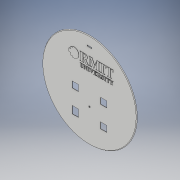
# Autodesk Inventor part: Cover
Saved by Autodesk Inventor 2018 (Build 220112000, 112)
## iProperties
Created: 2017-08-02
Part Number: Cover
Material: Generic
Document SubType Name: Modeling
Designer: Akram Al-Hourani
Density: 1 g/cm^3
Appearance: Default
Author: Akram Al-Hourani
Autodesk Inventor part; units mm, degrees
(part 1 of 2)
ref_plane "YZ Plane" through (0, 0, 0) normal (1, 0, 0) x (0, 1, 0)
ref_plane "XZ Plane" through (0, 0, 0) normal (0, 1, 0) x (-1, 0, 0)
ref_plane "XY Plane" through (0, 0, 0) normal (0, 0, 1) x (1, 0, 0)
sketch "Sketch1" plane through (0, 0, 0) normal (0, 0, 1) x (1, 0, 0)
  circle A0 centre (0, 0) radius 200
  circle A1 centre (0, 0) radius 194.25
  line L0 (-73, -28) -> (-47, -28)
  line L1 (-47, -28) -> (-47, -2)
  line L2 (-47, -2) -> (-73, -2)
  line L3 (-73, -2) -> (-73, -28)
  line L4 (-73, -28) -> (-47, -2) construction
  line L5 (-47, -28) -> (-73, -2) construction
  line L6 (47, -118) -> (73, -118)
  line L7 (73, -118) -> (73, -92)
  line L8 (73, -92) -> (47, -92)
  line L9 (47, -92) -> (47, -118)
  line L10 (47, -118) -> (73, -92) construction
  line L11 (73, -118) -> (47, -92) construction
  line L12 (47, -28) -> (73, -28)
  line L13 (73, -28) -> (73, -2)
  line L14 (73, -2) -> (47, -2)
  line L15 (47, -2) -> (47, -28)
  line L16 (47, -28) -> (73, -2) construction
  line L17 (73, -28) -> (47, -2) construction
  circle A2 centre (0, 0) radius 191.25
  line L18 (-103.842, 143.0933) -> (109.0153, 143.0933) construction
  line L19 (109.0153, 143.0933) -> (109.0153, 47.711) construction
  line L20 (109.0153, 47.711) -> (-103.842, 47.711) construction
  line L21 (-103.842, 47.711) -> (-103.842, 143.0933) construction
  line L22 (-70.0209, 127.2546) -> (-70.0209, 122.8615)
  line L23 (-70.0209, 122.8615) -> (-78.9535, 122.8615)
  line L24 (-78.9535, 122.8615) -> (-78.9535, 113.7335)
  line L25 (-78.9535, 113.7335) -> (-85.9337, 113.7335)
  line L26 (-85.9337, 113.7335) -> (-85.9337, 100.2125)
  line L27 (-85.9337, 100.2125) -> (-78.9535, 100.2125)
  line L28 (-78.9535, 100.2125) -> (-78.9535, 90.9382)
  line L29 (-78.9535, 90.9382) -> (-70.0209, 90.9382)
  line L30 (-70.0209, 90.9382) -> (-70.0209, 86.5939)
  line L31 (-70.0209, 86.5939) -> (-63.7485, 86.5939)
  line L32 (-70.0209, 127.2546) -> (-63.7485, 127.2546)
  arc A3 (-63.7485, 86.5939) -> (-63.7485, 127.2546) centre (-64.7193, 106.9242) ccw
  line L33 (-41.3776, 125.1847) -> (92.2863, 125.1847) construction
  line L34 (92.2863, 125.1847) -> (92.2863, 80.3812) construction
  line L35 (92.2863, 80.3812) -> (-41.3776, 80.3812) construction
  line L36 (-41.3776, 80.3812) -> (-41.3776, 125.1847) construction
  line L37 (-40.2575, 83.3681) -> (113.1946, 83.3681) construction
  line L38 (113.1946, 83.3681) -> (113.1946, 53.1257) construction
  line L39 (113.1946, 53.1257) -> (-40.2575, 53.1257) construction
  line L40 (-40.2575, 53.1257) -> (-40.2575, 83.3681) construction
  line L41 (-10, 156.8645) -> (10, 156.8645)
  line L42 (10, 156.8645) -> (10, 161.8645)
  line L43 (10, 161.8645) -> (-10, 161.8645)
  line L44 (-10, 161.8645) -> (-10, 156.8645)
  line L45 (-10, 156.8645) -> (10, 161.8645) construction
  line L46 (10, 156.8645) -> (-10, 161.8645) construction
  line L47 (-60, -15) -> (60, -105) construction
  line L48 (-60, -15) -> (60, -15) construction
  line L49 (60, -15) -> (60, -105) construction
  line L50 (60, -105) -> (-60, -105) construction
  line L51 (-60, -105) -> (-60, -15) construction
  line L52 (-73, -118) -> (-47, -118)
  line L53 (-47, -118) -> (-47, -92)
  line L54 (-47, -92) -> (-73, -92)
  line L55 (-73, -92) -> (-73, -118)
  line L56 (-73, -118) -> (-47, -92) construction
  line L57 (-47, -118) -> (-73, -92) construction
  line L58 (60, -15) -> (-60, -105) construction
  line L59 (-73, -118) -> (-47, -118)
  line L60 (-47, -118) -> (-47, -123)
  line L61 (-47, -123) -> (-73, -123)
  line L62 (-73, -123) -> (-73, -118)
  circle A4 centre (0, -60) radius 1
  circle A5 centre (0, -60) radius 3
  line L63 (-27.3375, 106.1406) -> (-27.3375, 96.3326)
  spline S0 degree 2 poles (-27.3375, 96.3326) (-27.3375, 93.4731) (-26.6513, 92.0148) (-24.8784, 91.1283) (-22.4764, 91.1283) knots 0 0 0 1 2 3 3 3
  line L64 (-22.4764, 91.1283) -> (-22.4764, 90.1847)
  line L65 (-22.4764, 90.1847) -> (-40.4053, 90.1847)
  line L66 (-40.4053, 90.1847) -> (-40.4053, 91.1283)
  spline S1 degree 2 poles (-40.4053, 91.1283) (-37.9748, 91.1283) (-36.2305, 92.0434) (-35.5442, 93.4731) (-35.5442, 96.3326) knots 0 0 0 1 2 3 3 3
  line L67 (-35.5442, 96.3326) -> (-35.5442, 119.0368)
  spline S2 degree 2 poles (-35.5442, 119.0368) (-35.5442, 121.8963) (-36.2305, 123.3546) (-38.0034, 124.2411) (-40.4053, 124.2411) knots 0 0 0 1 2 3 3 3
  line L68 (-40.4053, 124.2411) -> (-40.4053, 125.1847)
  line L69 (-40.4053, 125.1847) -> (-24.1349, 125.1847)
  spline S3 degree 2 poles (-24.1349, 125.1847) (-17.7869, 125.1847) (-11.8964, 123.4404) (-8.179, 118.7223) (-8.179, 115.5483) knots 0 0 0 1 2 3 3 3
  spline S4 degree 2 poles (-8.179, 115.5483) (-8.179, 111.6594) (-10.9813, 109.143) knots 0 0 0 1 1 1
  spline S5 degree 2 poles (-10.9813, 109.143) (-12.7542, 107.5417) (-15.9568, 106.7411) knots 0 0 0 1 1 1
  line L70 (-15.9568, 106.7411) -> (-7.55, 94.8743)
  spline S6 degree 2 poles (-7.55, 94.8743) (-5.8915, 92.5581) (-5.1766, 92.0148) knots 0 0 0 1 1 1
  spline S7 degree 2 poles (-5.1766, 92.0148) (-4.1186, 91.2141) (-2.7174, 91.1283) knots 0 0 0 1 1 1
  line L71 (-2.7174, 91.1283) -> (-2.7174, 90.1847)
  line L72 (-2.7174, 90.1847) -> (-13.755, 90.1847)
  line L73 (-13.755, 90.1847) -> (-25.05, 106.1406)
  line L74 (-25.05, 106.1406) -> (-27.3375, 106.1406)
  line L75 (-27.3375, 123.2975) -> (-27.3375, 107.9707)
  line L76 (-27.3375, 107.9707) -> (-25.8792, 107.9707)
  spline S8 degree 2 poles (-25.8792, 107.9707) (-22.2763, 107.9707) (-18.7019, 109.286) (-16.6717, 112.7174) (-16.6717, 115.4911) knots 0 0 0 1 2 3 3 3
  spline S9 degree 2 poles (-16.6717, 115.4911) (-16.6717, 119.4658) (-20.4176, 123.2975) (-24.5638, 123.2975) knots 0 0 0 1 2 2 2
  line L77 (-24.5638, 123.2975) -> (-27.3375, 123.2975)
  line L78 (22.017, 102.1659) -> (31.5105, 125.1847)
  line L79 (31.5105, 125.1847) -> (45.7221, 125.1847)
  line L80 (45.7221, 125.1847) -> (45.7221, 124.2411)
  line L81 (45.7221, 124.2411) -> (44.5783, 124.2411)
  spline S10 degree 2 poles (44.5783, 124.2411) (43.0342, 124.2411) (42.1192, 123.6978) knots 0 0 0 1 1 1
  spline S11 degree 2 poles (42.1192, 123.6978) (41.4615, 123.3261) (41.0897, 122.4682) knots 0 0 0 1 1 1
  spline S12 degree 2 poles (41.0897, 122.4682) (40.8038, 121.8677) (40.8038, 119.237) knots 0 0 0 1 1 1
  line L82 (40.8038, 119.237) -> (40.8038, 96.161)
  spline S13 degree 2 poles (40.8038, 96.161) (40.8038, 93.4731) (41.3757, 92.1292) (43.12, 91.1283) (44.5783, 91.1283) knots 0 0 0 1 2 3 3 3
  line L83 (44.5783, 91.1283) -> (45.7221, 91.1283)
  line L84 (45.7221, 91.1283) -> (45.7221, 90.1847)
  line L85 (45.7221, 90.1847) -> (27.4786, 90.1847)
  line L86 (27.4786, 90.1847) -> (27.4786, 91.1283)
  line L87 (27.4786, 91.1283) -> (28.6224, 91.1283)
  spline S14 degree 2 poles (28.6224, 91.1283) (30.1665, 91.1283) (31.0816, 91.6716) knots 0 0 0 1 1 1
  spline S15 degree 2 poles (31.0816, 91.6716) (31.7393, 92.0434) (32.111, 92.9012) knots 0 0 0 1 1 1
  spline S16 degree 2 poles (32.111, 92.9012) (32.3969, 93.5303) (32.3969, 96.161) knots 0 0 0 1 1 1
  line L88 (32.3969, 96.161) -> (32.3969, 122.0965)
  line L89 (32.3969, 122.0965) -> (18.986, 90.1847)
  line L90 (18.986, 90.1847) -> (18.3569, 90.1847)
  line L91 (18.3569, 90.1847) -> (4.7172, 121.8677)
  line L92 (4.7172, 121.8677) -> (4.7172, 97.219)
  spline S17 degree 2 poles (4.7172, 97.219) (4.7172, 94.6455) (4.8602, 94.045) knots 0 0 0 1 1 1
  spline S18 degree 2 poles (4.8602, 94.045) (5.1747, 92.7582) (7.4337, 91.1283) (9.8357, 91.1283) knots 0 0 0 1 2 2 2
  line L93 (9.8357, 91.1283) -> (9.8357, 90.1847)
  line L94 (9.8357, 90.1847) -> (-2.1741, 90.1847)
  line L95 (-2.1741, 90.1847) -> (-2.1741, 91.1283)
  line L96 (-2.1741, 91.1283) -> (-1.8024, 91.1283)
  spline S19 degree 2 poles (-1.8024, 91.1283) (-0.63, 91.0997) (1.3716, 91.9004) (2.401, 93.2729) (2.687, 94.4739) knots 0 0 0 1 2 3 3 3
  spline S20 degree 2 poles (2.687, 94.4739) (2.7442, 94.7599) (2.7442, 97.1332) knots 0 0 0 1 1 1
  line L97 (2.7442, 97.1332) -> (2.7442, 119.237)
  spline S21 degree 2 poles (2.7442, 119.237) (2.7442, 121.8963) (2.1723, 123.2403) (0.428, 124.2411) (-1.0589, 124.2411) knots 0 0 0 1 2 3 3 3
  line L98 (-1.0589, 124.2411) -> (-2.1741, 124.2411)
  line L99 (-2.1741, 124.2411) -> (-2.1741, 125.1847)
  line L100 (-2.1741, 125.1847) -> (12.1804, 125.1847)
  line L101 (12.1804, 125.1847) -> (22.017, 102.1659)
  line L102 (65.9958, 91.1283) -> (65.9958, 90.1847)
  line L103 (65.9958, 90.1847) -> (47.7523, 90.1847)
  line L104 (47.7523, 90.1847) -> (47.7523, 91.1283)
  line L105 (47.7523, 91.1283) -> (48.9247, 91.1283)
  spline S22 degree 2 poles (48.9247, 91.1283) (50.4402, 91.1283) (51.3553, 91.6716) knots 0 0 0 1 1 1
  spline S23 degree 2 poles (51.3553, 91.6716) (52.013, 92.0434) (52.3847, 92.9012) knots 0 0 0 1 1 1
  spline S24 degree 2 poles (52.3847, 92.9012) (52.6706, 93.5303) (52.6706, 96.161) knots 0 0 0 1 1 1
  line L106 (52.6706, 96.161) -> (52.6706, 119.2084)
  spline S25 degree 2 poles (52.6706, 119.2084) (52.6706, 121.8963) (52.0987, 123.2403) (50.383, 124.2411) (48.9247, 124.2411) knots 0 0 0 1 2 3 3 3
  line L107 (48.9247, 124.2411) -> (47.7523, 124.2411)
  line L108 (47.7523, 124.2411) -> (47.7523, 125.1847)
  line L109 (47.7523, 125.1847) -> (65.9958, 125.1847)
  line L110 (65.9958, 125.1847) -> (65.9958, 124.2411)
  line L111 (65.9958, 124.2411) -> (64.852, 124.2411)
  spline S26 degree 2 poles (64.852, 124.2411) (63.3365, 124.2411) (62.4214, 123.6978) knots 0 0 0 1 1 1
  spline S27 degree 2 poles (62.4214, 123.6978) (61.7352, 123.3261) (61.3634, 122.4682) knots 0 0 0 1 1 1
  spline S28 degree 2 poles (61.3634, 122.4682) (61.0775, 121.8391) (61.0775, 119.2084) knots 0 0 0 1 1 1
  line L112 (61.0775, 119.2084) -> (61.0775, 96.161)
  spline S29 degree 2 poles (61.0775, 96.161) (61.0775, 93.4731) (61.678, 92.1292) (63.3937, 91.1283) (64.852, 91.1283) knots 0 0 0 1 2 3 3 3
  line L113 (64.852, 91.1283) -> (65.9958, 91.1283)
  line L114 (100.6527, 125.1847) -> (100.6527, 115.7198)
  line L115 (100.6527, 115.7198) -> (99.709, 115.7198)
  spline S30 degree 2 poles (99.709, 115.7198) (98.8798, 119.0082) (96.8781, 121.8677) (95.1339, 122.7256) knots 0 0 0 1 2 2 2
  spline S31 degree 2 poles (95.1339, 122.7256) (94.1616, 123.1831) (91.7025, 123.1831) knots 0 0 0 1 1 1
  line L116 (91.7025, 123.1831) -> (89.1004, 123.1831)
  line L117 (89.1004, 123.1831) -> (89.1004, 96.161)
  spline S32 degree 2 poles (89.1004, 96.161) (89.1004, 93.4731) (89.7009, 92.1292) (91.4165, 91.1283) (92.9035, 91.1283) knots 0 0 0 1 2 3 3 3
  line L118 (92.9035, 91.1283) -> (94.0759, 91.1283)
  line L119 (94.0759, 91.1283) -> (94.0759, 90.1847)
  line L120 (94.0759, 90.1847) -> (75.7752, 90.1847)
  line L121 (75.7752, 90.1847) -> (75.7752, 91.1283)
  line L122 (75.7752, 91.1283) -> (76.919, 91.1283)
  spline S33 degree 2 poles (76.919, 91.1283) (78.4345, 91.1283) (79.3496, 91.6716) knots 0 0 0 1 1 1
  spline S34 degree 2 poles (79.3496, 91.6716) (80.0358, 92.0434) (80.4076, 92.9012) knots 0 0 0 1 1 1
  spline S35 degree 2 poles (80.4076, 92.9012) (80.6935, 93.5303) (80.6935, 96.161) knots 0 0 0 1 1 1
  line L123 (80.6935, 96.161) -> (80.6935, 123.1831)
  line L124 (80.6935, 123.1831) -> (78.1486, 123.1831)
  spline S36 degree 2 poles (78.1486, 123.1831) (74.6028, 123.1831) (73.0015, 121.6962) knots 0 0 0 1 1 1
  spline S37 degree 2 poles (73.0015, 121.6962) (70.7425, 119.5801) (70.142, 115.7198) knots 0 0 0 1 1 1
  line L125 (70.142, 115.7198) -> (69.1984, 115.7198)
  line L126 (69.1984, 115.7198) -> (69.1984, 125.1847)
  line L127 (69.1984, 125.1847) -> (100.6527, 125.1847)
  line L128 (-39.7305, 83.0249) -> (-31.9854, 83.0249)
  line L129 (-31.9854, 83.0249) -> (-31.9854, 82.6205)
  line L130 (-31.9854, 82.6205) -> (-32.3776, 82.6205)
  spline S38 degree 2 poles (-32.3776, 82.6205) (-33.2477, 82.6205) (-33.8972, 82.2529) (-34.1791, 81.6156) (-34.1791, 80.3289) knots 0 0 0 1 2 3 3 3
  line L131 (-34.1791, 80.3289) -> (-34.1791, 72.9882)
  spline S39 degree 2 poles (-34.1791, 72.9882) (-34.1791, 70.9784) (-33.5663, 69.6671) (-32.1815, 68.8093) (-31.1153, 68.8093) knots 0 0 0 1 2 3 3 3
  spline S40 degree 2 poles (-31.1153, 68.8093) (-29.9021, 68.8093) (-28.1864, 69.8999) (-27.3286, 71.824) (-27.3286, 74.2137) knots 0 0 0 1 2 3 3 3
  line L132 (-27.3286, 74.2137) -> (-27.3286, 80.3289)
  spline S41 degree 2 poles (-27.3286, 80.3289) (-27.3286, 81.3338) (-27.7452, 82.2039) (-28.0639, 82.3632) knots 0 0 0 1 2 2 2
  spline S42 degree 2 poles (-28.0639, 82.3632) (-28.5663, 82.6205) (-29.4732, 82.6205) knots 0 0 0 1 1 1
  line L133 (-29.4732, 82.6205) -> (-29.4732, 83.0249)
  line L134 (-29.4732, 83.0249) -> (-24.2893, 83.0249)
  line L135 (-24.2893, 83.0249) -> (-24.2893, 82.6205)
  line L136 (-24.2893, 82.6205) -> (-24.5957, 82.6205)
  spline S43 degree 2 poles (-24.5957, 82.6205) (-25.233, 82.6205) (-26.0663, 82.1058) (-26.2501, 81.6034) knots 0 0 0 1 2 2 2
  spline S44 degree 2 poles (-26.2501, 81.6034) (-26.3972, 81.248) (-26.3972, 80.3289) knots 0 0 0 1 1 1
  line L137 (-26.3972, 80.3289) -> (-26.3972, 74.6303)
  spline S45 degree 2 poles (-26.3972, 74.6303) (-26.3972, 71.9955) (-27.0957, 69.6549) (-29.7918, 67.6818) (-32.1325, 67.6818) knots 0 0 0 1 2 3 3 3
  spline S46 degree 2 poles (-32.1325, 67.6818) (-34.081, 67.6818) (-35.1349, 68.1965) knots 0 0 0 1 1 1
  spline S47 degree 2 poles (-35.1349, 68.1965) (-36.581, 68.9073) (-37.782, 71.1254) (-37.782, 72.9882) knots 0 0 0 1 2 2 2
  line L138 (-37.782, 72.9882) -> (-37.782, 80.3289)
  spline S48 degree 2 poles (-37.782, 80.3289) (-37.782, 81.6279) (-38.0639, 82.2529) (-38.7746, 82.6328) (-39.7305, 82.6205) knots 0 0 0 1 2 3 3 3
  line L139 (-39.7305, 82.6205) -> (-39.7305, 83.0249)
  line L140 (-18.2599, 83.0249) -> (-10.858, 73.7235)
  line L141 (-10.858, 73.7235) -> (-10.858, 80.1696)
  spline S49 degree 2 poles (-10.858, 80.1696) (-10.858, 81.5176) (-11.2501, 81.9955) knots 0 0 0 1 1 1
  spline S50 degree 2 poles (-11.2501, 81.9955) (-11.7771, 82.645) (-13.0271, 82.6205) knots 0 0 0 1 1 1
  line L142 (-13.0271, 82.6205) -> (-13.0271, 83.0249)
  line L143 (-13.0271, 83.0249) -> (-8.0639, 83.0249)
  line L144 (-8.0639, 83.0249) -> (-8.0639, 82.6205)
  spline S51 degree 2 poles (-8.0639, 82.6205) (-9.0197, 82.498) (-9.6692, 82.1058) (-10.0369, 81.2357) (-10.0369, 80.1696) knots 0 0 0 1 2 3 3 3
  line L145 (-10.0369, 80.1696) -> (-10.0369, 67.6818)
  line L146 (-10.0369, 67.6818) -> (-10.4168, 67.6818)
  line L147 (-10.4168, 67.6818) -> (-20.5639, 80.1818)
  line L148 (-20.5639, 80.1818) -> (-20.5639, 70.6352)
  spline S52 degree 2 poles (-20.5639, 70.6352) (-20.5639, 69.3362) (-19.3751, 68.4294) (-18.6153, 68.4294) knots 0 0 0 1 2 2 2
  line L149 (-18.6153, 68.4294) -> (-18.2599, 68.4294)
  line L150 (-18.2599, 68.4294) -> (-18.2599, 68.0249)
  line L151 (-18.2599, 68.0249) -> (-23.5908, 68.0249)
  line L152 (-23.5908, 68.0249) -> (-23.5908, 68.4294)
  spline S53 degree 2 poles (-23.5908, 68.4294) (-22.3531, 68.4416) (-21.3727, 69.4343) (-21.3727, 70.6352) knots 0 0 0 1 2 2 2
  line L153 (-21.3727, 70.6352) -> (-21.3727, 81.2235)
  line L154 (-21.3727, 81.2235) -> (-21.6913, 81.6156)
  spline S54 degree 2 poles (-21.6913, 81.6156) (-22.1692, 82.2161) (-22.8923, 82.596) (-23.5786, 82.6205) knots 0 0 0 1 2 2 2
  line L155 (-23.5786, 82.6205) -> (-23.5786, 83.0249)
  line L156 (-23.5786, 83.0249) -> (-18.2599, 83.0249)
  line L157 (0.7352, 68.4294) -> (0.7352, 68.0249)
  line L158 (0.7352, 68.0249) -> (-7.0835, 68.0249)
  line L159 (-7.0835, 68.0249) -> (-7.0835, 68.4294)
  line L160 (-7.0835, 68.4294) -> (-6.581, 68.4294)
  spline S55 degree 2 poles (-6.581, 68.4294) (-5.9315, 68.4294) (-5.5393, 68.6622) knots 0 0 0 1 1 1
  spline S56 degree 2 poles (-5.5393, 68.6622) (-5.2575, 68.8215) (-5.0982, 69.1892) knots 0 0 0 1 1 1
  spline S57 degree 2 poles (-5.0982, 69.1892) (-4.9756, 69.4588) (-4.9756, 70.5862) knots 0 0 0 1 1 1
  line L161 (-4.9756, 70.5862) -> (-4.9756, 80.4637)
  spline S58 degree 2 poles (-4.9756, 80.4637) (-4.9756, 81.6156) (-5.2207, 82.1916) (-5.956, 82.6205) (-6.581, 82.6205) knots 0 0 0 1 2 3 3 3
  line L162 (-6.581, 82.6205) -> (-7.0835, 82.6205)
  line L163 (-7.0835, 82.6205) -> (-7.0835, 83.0249)
  line L164 (-7.0835, 83.0249) -> (0.7352, 83.0249)
  line L165 (0.7352, 83.0249) -> (0.7352, 82.6205)
  line L166 (0.7352, 82.6205) -> (0.245, 82.6205)
  spline S59 degree 2 poles (0.245, 82.6205) (-0.4045, 82.6205) (-0.7967, 82.3877) knots 0 0 0 1 1 1
  spline S60 degree 2 poles (-0.7967, 82.3877) (-1.0908, 82.2284) (-1.2501, 81.8607) knots 0 0 0 1 1 1
  spline S61 degree 2 poles (-1.2501, 81.8607) (-1.3727, 81.5911) (-1.3727, 80.4637) knots 0 0 0 1 1 1
  line L167 (-1.3727, 80.4637) -> (-1.3727, 70.5862)
  spline S62 degree 2 poles (-1.3727, 70.5862) (-1.3727, 69.4343) (-1.1153, 68.8583) (-0.38, 68.4294) (0.245, 68.4294) knots 0 0 0 1 2 3 3 3
  line L168 (0.245, 68.4294) -> (0.7352, 68.4294)
  line L169 (17.4141, 83.0249) -> (17.4141, 82.6205)
  spline S63 degree 2 poles (17.4141, 82.6205) (16.593, 82.4857) (15.9558, 81.7504) knots 0 0 0 1 1 1
  spline S64 degree 2 poles (15.9558, 81.7504) (15.4901, 81.1867) (14.5709, 79.1401) knots 0 0 0 1 1 1
  line L170 (14.5709, 79.1401) -> (9.3994, 67.6818)
  line L171 (9.3994, 67.6818) -> (9.0317, 67.6818)
  line L172 (9.0317, 67.6818) -> (3.9092, 79.6181)
  spline S65 degree 2 poles (3.9092, 79.6181) (2.9778, 81.7749) (2.3528, 82.5225) (1.4827, 82.6205) knots 0 0 0 1 2 2 2
  line L173 (1.4827, 82.6205) -> (1.4827, 83.0249)
  line L174 (1.4827, 83.0249) -> (8.6518, 83.0249)
  line L175 (8.6518, 83.0249) -> (8.6518, 82.6205)
  line L176 (8.6518, 82.6205) -> (8.4067, 82.6205)
  spline S66 degree 2 poles (8.4067, 82.6205) (7.4386, 82.6205) (7.0832, 82.3754) knots 0 0 0 1 1 1
  spline S67 degree 2 poles (7.0832, 82.3754) (6.8259, 82.2039) (6.8259, 81.8852) knots 0 0 0 1 1 1
  spline S68 degree 2 poles (6.8259, 81.8852) (6.8259, 81.6892) (6.9974, 81.1499) (7.5121, 79.9612) knots 0 0 0 1 2 2 2
  line L177 (7.5121, 79.9612) -> (10.7107, 72.498)
  line L178 (10.7107, 72.498) -> (13.6763, 79.1524)
  spline S69 degree 2 poles (13.6763, 79.1524) (14.2033, 80.3534) (14.4484, 81.1622) (14.4484, 81.4563) knots 0 0 0 1 2 2 2
  spline S70 degree 2 poles (14.4484, 81.4563) (14.4484, 81.7872) (14.093, 82.3019) (13.7499, 82.4367) knots 0 0 0 1 2 2 2
  spline S71 degree 2 poles (13.7499, 82.4367) (13.2719, 82.6205) (12.4876, 82.6205) knots 0 0 0 1 1 1
  line L179 (12.4876, 82.6205) -> (12.4876, 83.0249)
  line L180 (12.4876, 83.0249) -> (17.4141, 83.0249)
  line L181 (23.8111, 82.1671) -> (23.8111, 76.0642)
  line L182 (23.8111, 76.0642) -> (24.1175, 76.0642)
  spline S72 degree 2 poles (24.1175, 76.0642) (25.5513, 76.0642) (26.8381, 77.8534) (27.0219, 79.6058) knots 0 0 0 1 2 2 2
  line L183 (27.0219, 79.6058) -> (27.4263, 79.6058)
  line L184 (27.4263, 79.6058) -> (27.4263, 71.7504)
  line L185 (27.4263, 71.7504) -> (27.0219, 71.7504)
  spline S73 degree 2 poles (27.0219, 71.7504) (26.8871, 73.0372) (26.0293, 74.6671) (24.8896, 75.2308) (23.8111, 75.2308) knots 0 0 0 1 2 3 3 3
  line L186 (23.8111, 75.2308) -> (23.8111, 71.0029)
  spline S74 degree 2 poles (23.8111, 71.0029) (23.8111, 69.7651) (24.0195, 69.2137) (24.5955, 68.8583) (25.245, 68.8583) knots 0 0 0 1 2 3 3 3
  line L187 (25.245, 68.8583) -> (26.1396, 68.8583)
  spline S75 degree 2 poles (26.1396, 68.8583) (28.2474, 68.8583) (30.7842, 70.8068) (31.3357, 72.7921) knots 0 0 0 1 2 2 2
  line L188 (31.3357, 72.7921) -> (31.7401, 72.7921)
  line L189 (31.7401, 72.7921) -> (31.066, 68.0249)
  line L190 (31.066, 68.0249) -> (18.1004, 68.0249)
  line L191 (18.1004, 68.0249) -> (18.1004, 68.4294)
  line L192 (18.1004, 68.4294) -> (18.6028, 68.4294)
  spline S76 degree 2 poles (18.6028, 68.4294) (19.2523, 68.4294) (19.6445, 68.6622) knots 0 0 0 1 1 1
  spline S77 degree 2 poles (19.6445, 68.6622) (19.9263, 68.8215) (20.0857, 69.1892) knots 0 0 0 1 1 1
  spline S78 degree 2 poles (20.0857, 69.1892) (20.2082, 69.4588) (20.2082, 70.5862) knots 0 0 0 1 1 1
  line L193 (20.2082, 70.5862) -> (20.2082, 80.4637)
  spline S79 degree 2 poles (20.2082, 80.4637) (20.2082, 81.4808) (20.1592, 81.7137) knots 0 0 0 1 1 1
  spline S80 degree 2 poles (20.1592, 81.7137) (20.0366, 82.1058) (19.7425, 82.3142) knots 0 0 0 1 1 1
  spline S81 degree 2 poles (19.7425, 82.3142) (19.3259, 82.6205) (18.6028, 82.6205) knots 0 0 0 1 1 1
  line L194 (18.6028, 82.6205) -> (18.1004, 82.6205)
  line L195 (18.1004, 82.6205) -> (18.1004, 83.0249)
  line L196 (18.1004, 83.0249) -> (30.6616, 83.0249)
  line L197 (30.6616, 83.0249) -> (30.6616, 78.5887)
  line L198 (30.6616, 78.5887) -> (30.2572, 78.5887)
  spline S82 degree 2 poles (30.2572, 78.5887) (29.9386, 80.2186) (28.7621, 81.6401) (27.6959, 81.971) knots 0 0 0 1 2 2 2
  spline S83 degree 2 poles (27.6959, 81.971) (27.0832, 82.1671) (25.3675, 82.1671) knots 0 0 0 1 1 1
  line L199 (25.3675, 82.1671) -> (23.8111, 82.1671)
  line L200 (38.7744, 74.8632) -> (38.7744, 70.6598)
  spline S84 degree 2 poles (38.7744, 70.6598) (38.7744, 69.4343) (39.0685, 68.8093) (39.8283, 68.4294) (40.8577, 68.4294) knots 0 0 0 1 2 3 3 3
  line L201 (40.8577, 68.4294) -> (40.8577, 68.0249)
  line L202 (40.8577, 68.0249) -> (33.1739, 68.0249)
  line L203 (33.1739, 68.0249) -> (33.1739, 68.4294)
  spline S85 degree 2 poles (33.1739, 68.4294) (34.2156, 68.4294) (34.9631, 68.8215) (35.2572, 69.4343) (35.2572, 70.6598) knots 0 0 0 1 2 3 3 3
  line L204 (35.2572, 70.6598) -> (35.2572, 80.3901)
  spline S86 degree 2 poles (35.2572, 80.3901) (35.2572, 81.6156) (34.9631, 82.2406) (34.2033, 82.6205) (33.1739, 82.6205) knots 0 0 0 1 2 3 3 3
  line L205 (33.1739, 82.6205) -> (33.1739, 83.0249)
  line L206 (33.1739, 83.0249) -> (40.1469, 83.0249)
  spline S87 degree 2 poles (40.1469, 83.0249) (42.8675, 83.0249) (45.392, 82.2774) (46.9852, 80.2553) (46.9852, 78.895) knots 0 0 0 1 2 3 3 3
  spline S88 degree 2 poles (46.9852, 78.895) (46.9852, 77.2284) (45.7842, 76.1499) knots 0 0 0 1 1 1
  spline S89 degree 2 poles (45.7842, 76.1499) (45.0244, 75.4637) (43.6518, 75.1205) knots 0 0 0 1 1 1
  line L207 (43.6518, 75.1205) -> (47.2548, 70.0348)
  spline S90 degree 2 poles (47.2548, 70.0348) (47.9656, 69.0421) (48.2719, 68.8093) knots 0 0 0 1 1 1
  spline S91 degree 2 poles (48.2719, 68.8093) (48.7254, 68.4661) (49.3259, 68.4294) knots 0 0 0 1 1 1
  line L208 (49.3259, 68.4294) -> (49.3259, 68.0249)
  line L209 (49.3259, 68.0249) -> (44.5955, 68.0249)
  line L210 (44.5955, 68.0249) -> (39.7548, 74.8632)
  line L211 (39.7548, 74.8632) -> (38.7744, 74.8632)
  line L212 (38.7744, 82.2161) -> (38.7744, 75.6475)
  line L213 (38.7744, 75.6475) -> (39.3994, 75.6475)
  spline S92 degree 2 poles (39.3994, 75.6475) (40.9435, 75.6475) (42.4754, 76.2112) (43.3455, 77.6818) (43.3455, 78.8705) knots 0 0 0 1 2 3 3 3
  spline S93 degree 2 poles (43.3455, 78.8705) (43.3455, 80.574) (41.7401, 82.2161) (39.9631, 82.2161) knots 0 0 0 1 2 2 2
  line L214 (39.9631, 82.2161) -> (38.7744, 82.2161)
  line L215 (59.7548, 83.3681) -> (59.8773, 78.3681)
  line L216 (59.8773, 78.3681) -> (59.4239, 78.3681)
  spline S94 degree 2 poles (59.4239, 78.3681) (59.1053, 80.2431) (56.5808, 82.5348) (55.1224, 82.5348) knots 0 0 0 1 2 2 2
  spline S95 degree 2 poles (55.1224, 82.5348) (53.995, 82.5348) (52.6714, 81.3338) (52.6714, 80.5495) knots 0 0 0 1 2 2 2
  spline S96 degree 2 poles (52.6714, 80.5495) (52.6714, 80.047) (52.9043, 79.6671) knots 0 0 0 1 1 1
  spline S97 degree 2 poles (52.9043, 79.6671) (53.2229, 79.1401) (53.9337, 78.6377) knots 0 0 0 1 1 1
  spline S98 degree 2 poles (53.9337, 78.6377) (54.4607, 78.27) (56.3479, 77.3387) knots 0 0 0 1 1 1
  spline S99 degree 2 poles (56.3479, 77.3387) (58.9827, 76.0519) (59.9018, 74.8999) knots 0 0 0 1 1 1
  spline S100 degree 2 poles (59.9018, 74.8999) (60.8087, 73.748) (60.8087, 72.2651) knots 0 0 0 1 1 1
  spline S101 degree 2 poles (60.8087, 72.2651) (60.8087, 70.3901) (57.8798, 67.6818) (55.6126, 67.6818) knots 0 0 0 1 2 2 2
  spline S102 degree 2 poles (55.6126, 67.6818) (54.9018, 67.6818) (53.6396, 67.9637) (52.6959, 68.3681) knots 0 0 0 1 2 2 2
  spline S103 degree 2 poles (52.6959, 68.3681) (52.1567, 68.5887) (51.8136, 68.5887) knots 0 0 0 1 1 1
  spline S104 degree 2 poles (51.8136, 68.5887) (51.5317, 68.5887) (50.8822, 68.1352) (50.6861, 67.6818) knots 0 0 0 1 2 2 2
  line L217 (50.6861, 67.6818) -> (50.2817, 67.6818)
  line L218 (50.2817, 67.6818) -> (50.2817, 73.3436)
  line L219 (50.2817, 73.3436) -> (50.6861, 73.3436)
  spline S105 degree 2 poles (50.6861, 73.3436) (51.1763, 70.9539) (53.9582, 68.4539) (55.5636, 68.4539) knots 0 0 0 1 2 2 2
  spline S106 degree 2 poles (55.5636, 68.4539) (56.8013, 68.4539) (58.2719, 69.8019) (58.2719, 70.6965) knots 0 0 0 1 2 2 2
  spline S107 degree 2 poles (58.2719, 70.6965) (58.2719, 71.2235) (57.7082, 72.2284) (56.5562, 73.123) (55.0857, 73.8338) knots 0 0 0 1 2 3 3 3
  spline S108 degree 2 poles (55.0857, 73.8338) (53.0391, 74.8387) (51.2499, 76.2602) (50.294, 78.0004) (50.294, 79.0544) knots 0 0 0 1 2 3 3 3
  spline S109 degree 2 poles (50.294, 79.0544) (50.294, 80.8436) (52.9288, 83.3681) (54.9263, 83.3681) knots 0 0 0 1 2 2 2
  spline S110 degree 2 poles (54.9263, 83.3681) (55.6616, 83.3681) (56.3479, 83.1965) knots 0 0 0 1 1 1
  spline S111 degree 2 poles (56.3479, 83.1965) (56.8626, 83.0617) (58.3577, 82.3387) (58.6641, 82.3387) knots 0 0 0 1 2 2 2
  spline S112 degree 2 poles (58.6641, 82.3387) (58.9459, 82.3387) (59.2768, 82.6941) (59.4239, 83.3681) knots 0 0 0 1 2 2 2
  line L220 (59.4239, 83.3681) -> (59.7548, 83.3681)
  line L221 (69.9876, 68.4294) -> (69.9876, 68.0249)
  line L222 (69.9876, 68.0249) -> (62.169, 68.0249)
  line L223 (62.169, 68.0249) -> (62.169, 68.4294)
  line L224 (62.169, 68.4294) -> (62.6714, 68.4294)
  spline S113 degree 2 poles (62.6714, 68.4294) (63.3209, 68.4294) (63.7131, 68.6622) knots 0 0 0 1 1 1
  spline S114 degree 2 poles (63.7131, 68.6622) (63.995, 68.8215) (64.1543, 69.1892) knots 0 0 0 1 1 1
  spline S115 degree 2 poles (64.1543, 69.1892) (64.2768, 69.4588) (64.2768, 70.5862) knots 0 0 0 1 1 1
  line L225 (64.2768, 70.5862) -> (64.2768, 80.4637)
  spline S116 degree 2 poles (64.2768, 80.4637) (64.2768, 81.6156) (64.0317, 82.1916) (63.2964, 82.6205) (62.6714, 82.6205) knots 0 0 0 1 2 3 3 3
  line L226 (62.6714, 82.6205) -> (62.169, 82.6205)
  line L227 (62.169, 82.6205) -> (62.169, 83.0249)
  line L228 (62.169, 83.0249) -> (69.9876, 83.0249)
  line L229 (69.9876, 83.0249) -> (69.9876, 82.6205)
  line L230 (69.9876, 82.6205) -> (69.4974, 82.6205)
  spline S117 degree 2 poles (69.4974, 82.6205) (68.8479, 82.6205) (68.4558, 82.3877) knots 0 0 0 1 1 1
  spline S118 degree 2 poles (68.4558, 82.3877) (68.1616, 82.2284) (68.0023, 81.8607) knots 0 0 0 1 1 1
  spline S119 degree 2 poles (68.0023, 81.8607) (67.8798, 81.5911) (67.8798, 80.4637) knots 0 0 0 1 1 1
  line L231 (67.8798, 80.4637) -> (67.8798, 70.5862)
  spline S120 degree 2 poles (67.8798, 70.5862) (67.8798, 69.4343) (68.1371, 68.8583) (68.8724, 68.4294) (69.4974, 68.4294) knots 0 0 0 1 2 3 3 3
  line L232 (69.4974, 68.4294) -> (69.9876, 68.4294)
  line L233 (84.8406, 83.0249) -> (84.8406, 78.9686)
  line L234 (84.8406, 78.9686) -> (84.4361, 78.9686)
  spline S121 degree 2 poles (84.4361, 78.9686) (84.0808, 80.3779) (83.2229, 81.6034) (82.4754, 81.971) knots 0 0 0 1 2 2 2
  spline S122 degree 2 poles (82.4754, 81.971) (82.0587, 82.1671) (81.0048, 82.1671) knots 0 0 0 1 1 1
  line L235 (81.0048, 82.1671) -> (79.8896, 82.1671)
  line L236 (79.8896, 82.1671) -> (79.8896, 70.5862)
  spline S123 degree 2 poles (79.8896, 70.5862) (79.8896, 69.4343) (80.1469, 68.8583) (80.8822, 68.4294) (81.5195, 68.4294) knots 0 0 0 1 2 3 3 3
  line L237 (81.5195, 68.4294) -> (82.0219, 68.4294)
  line L238 (82.0219, 68.4294) -> (82.0219, 68.0249)
  line L239 (82.0219, 68.0249) -> (74.1788, 68.0249)
  line L240 (74.1788, 68.0249) -> (74.1788, 68.4294)
  line L241 (74.1788, 68.4294) -> (74.669, 68.4294)
  spline S124 degree 2 poles (74.669, 68.4294) (75.3185, 68.4294) (75.7107, 68.6622) knots 0 0 0 1 1 1
  spline S125 degree 2 poles (75.7107, 68.6622) (76.0048, 68.8215) (76.1641, 69.1892) knots 0 0 0 1 1 1
  spline S126 degree 2 poles (76.1641, 69.1892) (76.2866, 69.4588) (76.2866, 70.5862) knots 0 0 0 1 1 1
  line L242 (76.2866, 70.5862) -> (76.2866, 82.1671)
  line L243 (76.2866, 82.1671) -> (75.1959, 82.1671)
  spline S127 degree 2 poles (75.1959, 82.1671) (73.6763, 82.1671) (72.9901, 81.5299) knots 0 0 0 1 1 1
  spline S128 degree 2 poles (72.9901, 81.5299) (72.0219, 80.623) (71.7646, 78.9686) knots 0 0 0 1 1 1
  line L244 (71.7646, 78.9686) -> (71.3602, 78.9686)
  line L245 (71.3602, 78.9686) -> (71.3602, 83.0249)
  line L246 (71.3602, 83.0249) -> (84.8406, 83.0249)
  line L247 (101.7523, 83.0249) -> (101.7523, 82.6205)
  spline S129 degree 2 poles (101.7523, 82.6205) (101.017, 82.5225) (100.6126, 82.1916) knots 0 0 0 1 1 1
  spline S130 degree 2 poles (100.6126, 82.1916) (100.0611, 81.7259) (98.8724, 79.6549) knots 0 0 0 1 1 1
  line L248 (98.8724, 79.6549) -> (95.6249, 74.2259)
  line L249 (95.6249, 74.2259) -> (95.6249, 70.5862)
  spline S131 degree 2 poles (95.6249, 70.5862) (95.6249, 69.422) (95.8577, 68.8583) (96.5808, 68.4294) (97.1812, 68.4294) knots 0 0 0 1 2 3 3 3
  line L250 (97.1812, 68.4294) -> (98.0268, 68.4294)
  line L251 (98.0268, 68.4294) -> (98.0268, 68.0249)
  line L252 (98.0268, 68.0249) -> (89.6077, 68.0249)
  line L253 (89.6077, 68.0249) -> (89.6077, 68.4294)
  line L254 (89.6077, 68.4294) -> (90.392, 68.4294)
  spline S132 degree 2 poles (90.392, 68.4294) (91.0538, 68.4294) (91.4459, 68.6622) knots 0 0 0 1 1 1
  spline S133 degree 2 poles (91.4459, 68.6622) (91.7278, 68.8215) (91.8994, 69.1892) knots 0 0 0 1 1 1
  spline S134 degree 2 poles (91.8994, 69.1892) (92.0219, 69.4588) (92.0219, 70.5862) knots 0 0 0 1 1 1
  line L255 (92.0219, 70.5862) -> (92.0219, 73.6009)
  line L256 (92.0219, 73.6009) -> (88.4925, 80.0348)
  spline S135 degree 2 poles (88.4925, 80.0348) (87.4386, 81.9343) (86.5685, 82.6083) (85.8577, 82.6205) knots 0 0 0 1 2 2 2
  line L257 (85.8577, 82.6205) -> (85.8577, 83.0249)
  line L258 (85.8577, 83.0249) -> (93.0268, 83.0249)
  line L259 (93.0268, 83.0249) -> (93.0268, 82.6205)
  line L260 (93.0268, 82.6205) -> (92.7082, 82.6205)
  spline S136 degree 2 poles (92.7082, 82.6205) (92.0587, 82.6205) (91.5317, 82.2406) (91.5317, 82.0323) knots 0 0 0 1 2 2 2
  spline S137 degree 2 poles (91.5317, 82.0323) (91.5317, 81.6279) (92.4263, 80.0225) knots 0 0 0 1 1 1
  line L261 (92.4263, 80.0225) -> (95.1469, 75.0715)
  line L262 (95.1469, 75.0715) -> (97.843, 79.5813)
  spline S138 degree 2 poles (97.843, 79.5813) (98.8479, 81.248) (98.8479, 81.7872) knots 0 0 0 1 1 1
  spline S139 degree 2 poles (98.8479, 81.7872) (98.8479, 82.0936) (98.566, 82.2897) knots 0 0 0 1 1 1
  spline S140 degree 2 poles (98.566, 82.2897) (98.1861, 82.5593) (97.1812, 82.6205) knots 0 0 0 1 1 1
  line L263 (97.1812, 82.6205) -> (97.1812, 83.0249)
  line L264 (97.1812, 83.0249) -> (101.7523, 83.0249)
  point P0 (60, -15)
  point P1 (60, -105)
  point P2 (60, -105)
  point P3 (0, 159.3645)
  dimension "d118" = 26
  dimension "d119" = 26
  dimension "d122" = 26
  dimension "d123" = 26
  dimension "d124" = 26
  dimension "d125" = 26
  dimension "d126" = 388.5
  dimension "d127" = 3
  dimension "d145" = 20
  dimension "d146" = 5
  dimension "d287" = 26
  dimension "d288" = 26
  dimension "d289" = 26
  dimension "d290" = 5
  dimension "d298" = 2
  dimension "d300" = 2
  constraints: 102 end point, 17 midpoint, 14 parallel, 14 perpendicular, 7 horizontal, 6 centre point, 4 point on line, 2 point on circle, 1 vertical, 6 other
  measures "d118" distance of L2.end L1.end
  measures "d119" distance of L1.end L0.end
  measures "d122" distance of L8.end L7.end
  measures "d123" distance of L7.end L6.end
  measures "d124" distance of L14.end L13.end
  measures "d125" distance of L13.end L12.end
  measures "d126" diameter of A1
  measures "d127" radial gap between concentric circles of A1 A2
  measures "d145" distance of L43.end L42.end
  measures "d146" distance of L42.end L41.end
  measures "d287" distance of L54.end L53.end
  measures "d288" distance of L53.end L52.end
  measures "d289" distance of L60.end L61.end
  measures "d290" distance of L59.end L60.end
  measures "d298" diameter of A4
  measures "d300" radial gap between concentric circles of A4 A5
extrude "Extrusion2" add sketch "Sketch1" against normal blind 5.5 contours A1
extrude "Extrusion3" add sketch "Sketch1" against normal blind 2.5 contours A0
fillet "Fillet1" radius 2.5 1 edges at (-200, 0, 0)
fillet "Fillet2" radius 1 1 edges at (-194.25, 0, -5.5)
extrude "Extrusion4" cut sketch "Sketch1" against normal blind 2.5 contours L44 L43 L42 L41
extrude "Extrusion5" add sketch "Sketch1" along normal blind 1 contours L32 A3 L31 L30 L29 L28 L27 L26 L25 L24 L23 L22
sketch "Sketch2" plane through (0, 0, 0) normal (0, 0, 1) x (1, 0, 0)
  circle A0 centre (0, 0) radius 200
  circle A1 centre (0, 0) radius 175 construction
  circle A2 centre (0, 0) radius 195
  line L0 (75, -3) -> (125, -3)
  line L1 (125, -3) -> (125, -117)
  line L2 (125, -117) -> (75, -117)
  line L3 (75, -117) -> (75, -3)
  line L4 (-125, -3) -> (-75, -3)
  line L5 (-75, -3) -> (-75, -117)
  line L6 (-75, -117) -> (-125, -117)
  line L7 (-125, -117) -> (-125, -3)
  line L8 (100, -60) -> (-100, -60) construction
  line L9 (-75, -3) -> (-125, -117) construction
  line L10 (-125, -3) -> (-75, -117) construction
  line L11 (75, -3) -> (125, -117) construction
  line L12 (125, -3) -> (75, -117) construction
  line L13 (100, -60) -> (4, -60) construction
  line L14 (-100, -60) -> (-4, -60) construction
  line L15 (4, -81.35) -> (100, -81.35) construction
  line L16 (100, -81.35) -> (100, -38.65) construction
  line L17 (100, -38.65) -> (4, -38.65) construction
  line L18 (4, -38.65) -> (4, -81.35) construction
  line L19 (4, -81.35) -> (100, -38.65) construction
  line L20 (100, -81.35) -> (4, -38.65) construction
  line L21 (-100.0669, -81.35) -> (-3.9331, -81.35) construction
  line L22 (-3.9331, -81.35) -> (-3.9331, -38.65) construction
  line L23 (-3.9331, -38.65) -> (-100.0669, -38.65) construction
  line L24 (-100.0669, -38.65) -> (-100.0669, -81.35) construction
  line L25 (-100.0669, -81.35) -> (-3.9331, -38.65) construction
  line L26 (-3.9331, -81.35) -> (-100.0669, -38.65) construction
  line L27 (0, 0) -> (0, -60) construction
  line L28 (-20, 130) -> (20, 130)
  line L29 (20, 130) -> (20, 170)
  line L30 (20, 170) -> (-20, 170)
  line L31 (-20, 170) -> (-20, 130)
  line L32 (-20, 130) -> (20, 170) construction
  line L33 (20, 130) -> (-20, 170) construction
  line L34 (0, -60) -> (0, 150) construction
  line L35 (0, 0) -> (0, 58) construction
  line L36 (0, 58) -> (-110, 58) construction
  line L37 (0, 58) -> (110, 58) construction
  line L38 (91.75, 24.75) -> (128.25, 24.75) construction
  line L39 (128.25, 24.75) -> (128.25, 91.25) construction
  line L40 (128.25, 91.25) -> (91.75, 91.25) construction
  line L41 (91.75, 91.25) -> (91.75, 24.75) construction
  line L42 (91.75, 24.75) -> (128.25, 91.25) construction
  line L43 (128.25, 24.75) -> (91.75, 91.25) construction
  line L44 (4, -38.65) -> (4, -26.65) construction
  line L45 (-3.9331, -81.35) -> (-3.9331, -93.35) construction
  line L46 (4, -26.65) -> (-3.9331, -26.65)
  line L47 (-3.9331, -26.65) -> (-3.9331, -93.35)
  line L48 (-3.9331, -93.35) -> (4, -93.35)
  line L49 (4, -93.35) -> (4, -26.65)
  line L50 (4, -26.65) -> (75, -26.65)
  line L51 (75, -26.65) -> (75, -38.65)
  line L52 (75, -38.65) -> (4, -38.65)
  line L53 (4, -38.65) -> (4, -26.65)
  line L54 (75, -81.35) -> (4, -81.35)
  line L55 (4, -81.35) -> (4, -93.35)
  line L56 (4, -93.35) -> (75, -93.35)
  line L57 (75, -93.35) -> (75, -81.35)
  line L58 (-3.9331, -26.65) -> (-75, -26.65)
  line L59 (-75, -26.65) -> (-75, -38.65)
  line L60 (-75, -38.65) -> (-3.9331, -38.65)
  line L61 (-3.9331, -38.65) -> (-3.9331, -26.65)
  line L62 (-3.9331, -81.35) -> (-75, -81.35)
  line L63 (-75, -81.35) -> (-75, -93.35)
  line L64 (-75, -93.35) -> (-3.9331, -93.35)
  line L65 (-3.9331, -93.35) -> (-3.9331, -81.35)
  line L66 (4, -32.65) -> (56, -32.65) construction
  line L67 (-138.75, 1) -> (-81.25, 1) construction
  line L68 (-81.25, 1) -> (-81.25, 115) construction
  line L69 (-81.25, 115) -> (-138.75, 115) construction
  line L70 (-138.75, 115) -> (-138.75, 1) construction
  line L71 (-138.75, 1) -> (-81.25, 115) construction
  line L72 (-81.25, 1) -> (-138.75, 115) construction
  line L73 (-138.75, 115) -> (-123.75, 115)
  line L74 (-123.75, 115) -> (-123.75, 118)
  line L75 (-123.75, 118) -> (-138.75, 118)
  line L76 (-138.75, 118) -> (-138.75, 115)
  line L77 (-138.75, 118) -> (-141.75, 118)
  line L78 (-141.75, 118) -> (-141.75, 100)
  line L79 (-141.75, 100) -> (-138.75, 100)
  line L80 (-138.75, 100) -> (-138.75, 118)
  line L81 (-81.25, 115) -> (-96.25, 115)
  line L82 (-96.25, 115) -> (-96.25, 118)
  line L83 (-96.25, 118) -> (-81.25, 118)
  line L84 (-81.25, 118) -> (-81.25, 115)
  line L85 (-81.25, 118) -> (-78.25, 118)
  line L86 (-78.25, 118) -> (-78.25, 100)
  line L87 (-78.25, 100) -> (-81.25, 100)
  line L88 (-81.25, 100) -> (-81.25, 118)
  line L89 (-100, -60) -> (-150, -60) construction
  line L90 (-155, -70) -> (-145, -70)
  line L91 (-145, -70) -> (-145, -50)
  line L92 (-145, -50) -> (-155, -50)
  line L93 (-155, -50) -> (-155, -70)
  line L94 (-155, -70) -> (-145, -50) construction
  line L95 (-145, -70) -> (-155, -50) construction
  line L96 (100, -60) -> (150, -60) construction
  line L97 (145, -70) -> (155, -70)
  line L98 (155, -70) -> (155, -50)
  line L99 (155, -50) -> (145, -50)
  line L100 (145, -50) -> (145, -70)
  line L101 (145, -70) -> (155, -50) construction
  line L102 (155, -70) -> (145, -50) construction
  line L103 (91.75, 91.25) -> (101.75, 91.25)
  line L104 (101.75, 91.25) -> (101.75, 94.25)
  line L105 (101.75, 94.25) -> (91.75, 94.25)
  line L106 (91.75, 94.25) -> (91.75, 91.25)
  line L107 (128.25, 91.25) -> (118.25, 91.25)
  line L108 (118.25, 91.25) -> (118.25, 94.25)
  line L109 (118.25, 94.25) -> (128.25, 94.25)
  line L110 (128.25, 94.25) -> (128.25, 91.25)
  line L111 (91.75, 94.25) -> (88.75, 94.25)
  line L112 (88.75, 94.25) -> (88.75, 76.25)
  line L113 (88.75, 76.25) -> (91.75, 76.25)
  line L114 (91.75, 76.25) -> (91.75, 94.25)
  line L115 (128.25, 94.25) -> (131.25, 94.25)
  line L116 (131.25, 94.25) -> (131.25, 79.25)
  line L117 (131.25, 79.25) -> (128.25, 79.25)
  line L118 (128.25, 79.25) -> (128.25, 94.25)
  line L119 (91.75, 24.75) -> (101.75, 24.75)
  line L120 (101.75, 24.75) -> (101.75, 21.75)
  line L121 (101.75, 21.75) -> (91.75, 21.75)
  line L122 (91.75, 21.75) -> (91.75, 24.75)
  line L123 (91.75, 21.75) -> (88.75, 21.75)
  line L124 (88.75, 21.75) -> (88.75, 39.75)
  line L125 (88.75, 39.75) -> (91.75, 39.75)
  line L126 (91.75, 39.75) -> (91.75, 21.75)
  line L127 (128.25, 24.75) -> (118.25, 24.75)
  line L128 (118.25, 24.75) -> (118.25, 21.75)
  line L129 (118.25, 21.75) -> (128.25, 21.75)
  line L130 (128.25, 21.75) -> (128.25, 24.75)
  line L131 (128.25, 21.75) -> (131.25, 21.75)
  line L132 (131.25, 21.75) -> (131.25, 39.75)
  line L133 (131.25, 39.75) -> (128.25, 39.75)
  line L134 (128.25, 39.75) -> (128.25, 21.75)
  line L135 (-13.65, 136.35) -> (13.65, 136.35) construction
  line L136 (13.65, 136.35) -> (13.65, 163.65) construction
  line L137 (13.65, 163.65) -> (-13.65, 163.65) construction
  line L138 (-13.65, 163.65) -> (-13.65, 136.35) construction
  line L139 (-13.65, 136.35) -> (13.65, 163.65) construction
  line L140 (13.65, 136.35) -> (-13.65, 163.65) construction
  circle A3 centre (-13.65, 163.65) radius 2.5
  circle A4 centre (13.65, 163.65) radius 2.5
  circle A5 centre (13.65, 136.35) radius 2.5
  circle A6 centre (-13.65, 136.35) radius 2.5
  line L141 (195, 0) -> (175, 0) construction
  line L142 (185, 0) -> (191, 0) construction
  line L143 (191, 12) -> (191, -12) construction
  line L144 (189, 12) -> (189, -12)
  line L145 (193, -12) -> (193, 12)
  arc A7 (193, 12) -> (189, 12) centre (191, 12) ccw
  arc A8 (189, -12) -> (193, -12) centre (191, -12) ccw
  line L146 (185, 0) -> (179, 0) construction
  line L147 (179, -12) -> (179, 12) construction
  line L148 (181, -12) -> (181, 12)
  line L149 (177, 12) -> (177, -12)
  arc A9 (177, -12) -> (181, -12) centre (179, -12) ccw
  arc A10 (181, 12) -> (177, 12) centre (179, 12) ccw
  line L150 (159.2865, -78.1077) -> (147.2865, -98.8923)
  line L151 (149.0185, -99.8923) -> (161.0185, -79.1077) construction
  line L152 (150.7506, -100.8923) -> (162.7506, -80.1077)
  arc A11 (162.7506, -80.1077) -> (159.2865, -78.1077) centre (161.0185, -79.1077) ccw
  arc A12 (147.2865, -98.8923) -> (150.7506, -100.8923) centre (149.0185, -99.8923) ccw
  line L153 (169.6788, -84.1077) -> (157.6788, -104.8923)
  line L154 (171.4109, -85.1077) -> (159.4109, -105.8923) construction
  line L155 (161.1429, -106.8923) -> (173.1429, -86.1077)
  arc A13 (173.1429, -86.1077) -> (169.6788, -84.1077) centre (171.4109, -85.1077) ccw
  arc A14 (157.6788, -104.8923) -> (161.1429, -106.8923) centre (159.4109, -105.8923) ccw
  line L156 (98.8923, -147.2865) -> (78.1077, -159.2865)
  line L157 (79.1077, -161.0185) -> (99.8923, -149.0185) construction
  line L158 (80.1077, -162.7506) -> (100.8923, -150.7506)
  arc A15 (100.8923, -150.7506) -> (98.8923, -147.2865) centre (99.8923, -149.0185) ccw
  arc A16 (78.1077, -159.2865) -> (80.1077, -162.7506) centre (79.1077, -161.0185) ccw
  line L159 (104.8923, -157.6788) -> (84.1077, -169.6788)
  line L160 (105.8923, -159.4109) -> (85.1077, -171.4109) construction
  line L161 (86.1077, -173.1429) -> (106.8923, -161.1429)
  arc A17 (106.8923, -161.1429) -> (104.8923, -157.6788) centre (105.8923, -159.4109) ccw
  arc A18 (84.1077, -169.6788) -> (86.1077, -173.1429) centre (85.1077, -171.4109) ccw
  line L162 (12, -177) -> (-12, -177)
  line L163 (-12, -179) -> (12, -179) construction
  line L164 (-12, -181) -> (12, -181)
  arc A19 (12, -181) -> (12, -177) centre (12, -179) ccw
  arc A20 (-12, -177) -> (-12, -181) centre (-12, -179) ccw
  line L165 (12, -189) -> (-12, -189)
  line L166 (12, -191) -> (-12, -191) construction
  line L167 (-12, -193) -> (12, -193)
  arc A21 (12, -193) -> (12, -189) centre (12, -191) ccw
  arc A22 (-12, -189) -> (-12, -193) centre (-12, -191) ccw
  line L168 (-78.1077, -159.2865) -> (-98.8923, -147.2865)
  line L169 (-99.8923, -149.0185) -> (-79.1077, -161.0185) construction
  line L170 (-100.8923, -150.7506) -> (-80.1077, -162.7506)
  arc A23 (-80.1077, -162.7506) -> (-78.1077, -159.2865) centre (-79.1077, -161.0185) ccw
  arc A24 (-98.8923, -147.2865) -> (-100.8923, -150.7506) centre (-99.8923, -149.0185) ccw
  line L171 (-84.1077, -169.6788) -> (-104.8923, -157.6788)
  line L172 (-85.1077, -171.4109) -> (-105.8923, -159.4109) construction
  line L173 (-106.8923, -161.1429) -> (-86.1077, -173.1429)
  arc A25 (-86.1077, -173.1429) -> (-84.1077, -169.6788) centre (-85.1077, -171.4109) ccw
  arc A26 (-104.8923, -157.6788) -> (-106.8923, -161.1429) centre (-105.8923, -159.4109) ccw
  line L174 (-147.2865, -98.8923) -> (-159.2865, -78.1077)
  line L175 (-161.0185, -79.1077) -> (-149.0185, -99.8923) construction
  line L176 (-162.7506, -80.1077) -> (-150.7506, -100.8923)
  arc A27 (-150.7506, -100.8923) -> (-147.2865, -98.8923) centre (-149.0185, -99.8923) ccw
  arc A28 (-159.2865, -78.1077) -> (-162.7506, -80.1077) centre (-161.0185, -79.1077) ccw
  line L177 (-157.6788, -104.8923) -> (-169.6788, -84.1077)
  line L178 (-159.4109, -105.8923) -> (-171.4109, -85.1077) construction
  line L179 (-173.1429, -86.1077) -> (-161.1429, -106.8923)
  arc A29 (-161.1429, -106.8923) -> (-157.6788, -104.8923) centre (-159.4109, -105.8923) ccw
  arc A30 (-169.6788, -84.1077) -> (-173.1429, -86.1077) centre (-171.4109, -85.1077) ccw
  line L180 (-177, -12) -> (-177, 12)
  line L181 (-179, 12) -> (-179, -12) construction
  line L182 (-181, 12) -> (-181, -12)
  arc A31 (-181, -12) -> (-177, -12) centre (-179, -12) ccw
  arc A32 (-177, 12) -> (-181, 12) centre (-179, 12) ccw
  line L183 (-189, -12) -> (-189, 12)
  line L184 (-191, -12) -> (-191, 12) construction
  line L185 (-193, 12) -> (-193, -12)
  arc A33 (-193, -12) -> (-189, -12) centre (-191, -12) ccw
  arc A34 (-189, 12) -> (-193, 12) centre (-191, 12) ccw
  line L186 (-159.2865, 78.1077) -> (-147.2865, 98.8923)
  line L187 (-149.0185, 99.8923) -> (-161.0185, 79.1077) construction
  line L188 (-150.7506, 100.8923) -> (-162.7506, 80.1077)
  arc A35 (-162.7506, 80.1077) -> (-159.2865, 78.1077) centre (-161.0185, 79.1077) ccw
  arc A36 (-147.2865, 98.8923) -> (-150.7506, 100.8923) centre (-149.0185, 99.8923) ccw
  line L189 (-169.6788, 84.1077) -> (-157.6788, 104.8923)
  line L190 (-171.4109, 85.1077) -> (-159.4109, 105.8923) construction
  line L191 (-161.1429, 106.8923) -> (-173.1429, 86.1077)
  arc A37 (-173.1429, 86.1077) -> (-169.6788, 84.1077) centre (-171.4109, 85.1077) ccw
  arc A38 (-157.6788, 104.8923) -> (-161.1429, 106.8923) centre (-159.4109, 105.8923) ccw
  line L192 (-98.8923, 147.2865) -> (-78.1077, 159.2865)
  line L193 (-79.1077, 161.0185) -> (-99.8923, 149.0185) construction
  line L194 (-80.1077, 162.7506) -> (-100.8923, 150.7506)
  arc A39 (-100.8923, 150.7506) -> (-98.8923, 147.2865) centre (-99.8923, 149.0185) ccw
  arc A40 (-78.1077, 159.2865) -> (-80.1077, 162.7506) centre (-79.1077, 161.0185) ccw
  line L195 (-104.8923, 157.6788) -> (-84.1077, 169.6788)
  line L196 (-105.8923, 159.4109) -> (-85.1077, 171.4109) construction
  line L197 (-86.1077, 173.1429) -> (-106.8923, 161.1429)
  arc A41 (-106.8923, 161.1429) -> (-104.8923, 157.6788) centre (-105.8923, 159.4109) ccw
  arc A42 (-84.1077, 169.6788) -> (-86.1077, 173.1429) centre (-85.1077, 171.4109) ccw
  line L198 (-12, 177) -> (12, 177)
  line L199 (12, 179) -> (-12, 179) construction
  line L200 (12, 181) -> (-12, 181)
  arc A43 (-12, 181) -> (-12, 177) centre (-12, 179) ccw
  arc A44 (12, 177) -> (12, 181) centre (12, 179) ccw
  line L201 (-12, 189) -> (12, 189)
  line L202 (-12, 191) -> (12, 191) construction
  line L203 (12, 193) -> (-12, 193)
  arc A45 (-12, 193) -> (-12, 189) centre (-12, 191) ccw
  arc A46 (12, 189) -> (12, 193) centre (12, 191) ccw
  line L204 (78.1077, 159.2865) -> (98.8923, 147.2865)
  line L205 (99.8923, 149.0185) -> (79.1077, 161.0185) construction
  line L206 (100.8923, 150.7506) -> (80.1077, 162.7506)
  arc A47 (80.1077, 162.7506) -> (78.1077, 159.2865) centre (79.1077, 161.0185) ccw
  arc A48 (98.8923, 147.2865) -> (100.8923, 150.7506) centre (99.8923, 149.0185) ccw
  line L207 (84.1077, 169.6788) -> (104.8923, 157.6788)
  line L208 (85.1077, 171.4109) -> (105.8923, 159.4109) construction
  line L209 (106.8923, 161.1429) -> (86.1077, 173.1429)
  arc A49 (86.1077, 173.1429) -> (84.1077, 169.6788) centre (85.1077, 171.4109) ccw
  arc A50 (104.8923, 157.6788) -> (106.8923, 161.1429) centre (105.8923, 159.4109) ccw
  line L210 (147.2865, 98.8923) -> (159.2865, 78.1077)
  line L211 (161.0185, 79.1077) -> (149.0185, 99.8923) construction
  line L212 (162.7506, 80.1077) -> (150.7506, 100.8923)
  arc A51 (150.7506, 100.8923) -> (147.2865, 98.8923) centre (149.0185, 99.8923) ccw
  arc A52 (159.2865, 78.1077) -> (162.7506, 80.1077) centre (161.0185, 79.1077) ccw
  line L213 (157.6788, 104.8923) -> (169.6788, 84.1077)
  line L214 (159.4109, 105.8923) -> (171.4109, 85.1077) construction
  line L215 (173.1429, 86.1077) -> (161.1429, 106.8923)
  arc A53 (161.1429, 106.8923) -> (157.6788, 104.8923) centre (159.4109, 105.8923) ccw
  arc A54 (169.6788, 84.1077) -> (173.1429, 86.1077) centre (171.4109, 85.1077) ccw
  line L216 (-72, 0) -> (-128, 0)
  line L217 (-128, 0) -> (-128, -120)
  line L218 (-128, -120) -> (-72, -120)
  line L219 (72, 0) -> (128, 0)
  line L220 (128, 0) -> (128, -120)
  line L221 (128, -120) -> (72, -120)
  line L222 (-72, 0) -> (-72, -26.65)
  line L223 (-75, -26.65) -> (-75, -3)
  line L224 (-72, -120) -> (-72, -93.35)
  line L225 (-75, -93.35) -> (-75, -117)
  line L226 (72, -38.65) -> (72, 0)
  line L227 (72, -120) -> (72, -81.35)
  circle A55 centre (0, 150) radius 40
  circle A56 centre (0, 150) radius 35
  line L228 (0, 0) -> (0, 47) construction
  line L229 (-76, -0.5) -> (76, -0.5) construction
  line L230 (76, -0.5) -> (76, 94.5) construction
  line L231 (76, 94.5) -> (-76, 94.5) construction
  line L232 (-76, 94.5) -> (-76, -0.5) construction
  line L233 (-76, -0.5) -> (76, 94.5) construction
  line L234 (76, -0.5) -> (-76, 94.5) construction
  line L235 (72, 0) -> (-72, 0)
  line L236 (-72, 0) -> (-72, -5)
  line L237 (-72, -5) -> (72, -5)
  line L238 (72, -5) -> (72, 0)
  line L239 (-76, 94.5) -> (-81, 94.5)
  line L240 (-81, 94.5) -> (-81, 1)
  line L241 (-81, 1) -> (-76, 1)
  line L242 (-76, 1) -> (-76, 94.5)
  line L243 (76, 94.5) -> (81, 94.5)
  line L244 (81, 94.5) -> (81, 0)
  line L245 (81, 0) -> (76, 0)
  line L246 (76, 0) -> (76, 94.5)
  line L247 (0, 94.5) -> (-30, 94.5) construction
  line L248 (-30, 94.5) -> (30, 94.5)
  line L249 (30, 94.5) -> (30, 111.5)
  line L250 (30, 111.5) -> (-30, 111.5)
  line L251 (-30, 111.5) -> (-30, 94.5)
  line L252 (4, -32.65) -> (30, -32.65) construction
  line L253 (30, -32.65) -> (17, -32.65) construction
  line L254 (30, -32.65) -> (43, -32.65) construction
  circle A57 centre (43, -32.65) radius 2.5
  circle A58 centre (17, -32.65) radius 2.5
  line L255 (-3.9331, -32.65) -> (-29.9331, -32.65) construction
  line L256 (-29.9331, -32.65) -> (-16.9331, -32.65) construction
  line L257 (-16.9331, -32.65) -> (-42.9331, -32.65) construction
  circle A59 centre (-16.9331, -32.65) radius 2.5